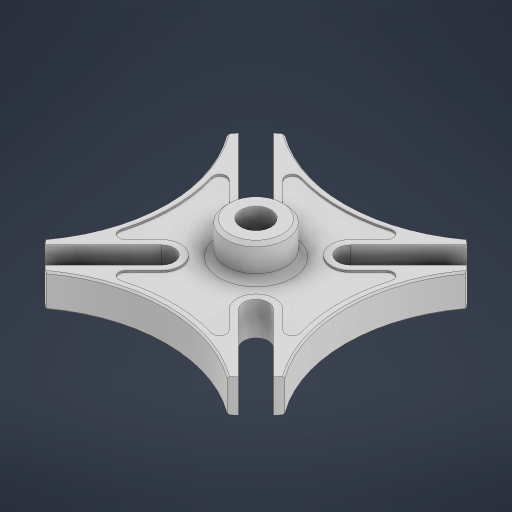
# Autodesk Inventor part: Malta cross
Saved by Autodesk Inventor 2023.2 (Build 272271000, 271)
## iProperties
Created: 2022-11-28
Part Number: Malta cross
Material: Generic
Document SubType Name: Modeling
Designer: iusti
Density: 1 g/cm^3
Appearance: Gunmetal - Antique Polished
Author: iusti
Autodesk Inventor part; units mm, degrees
ref_plane "YZ Plane" through (0, 0, 0) normal (1, 0, 0) x (0, 1, 0)
ref_plane "XZ Plane" through (0, 0, 0) normal (0, 1, 0) x (-1, 0, 0)
sketch "Sketch2" plane through (0, 0, 0) normal (0, 1, 0) x (-1, 0, 0)
  circle A0 centre (0, 0) radius 45 construction
  arc A1 (35.8767, 27.1636) -> (35.8767, -27.1636) centre (73, 0) ccw
  arc A2 (-27.1636, 35.8767) -> (27.1636, 35.8767) centre (0, 73) ccw
  arc A3 (-35.8767, -27.1636) -> (-35.8767, 27.1636) centre (-73, 0) ccw
  arc A4 (27.1636, -35.8767) -> (-27.1636, -35.8767) centre (0, -73) ccw
  circle A5 centre (0, 0) radius 20 construction
  line L0 (0, 0) -> (31.8198, -31.8198) construction
  line L1 (0, 0) -> (45, 0) construction
  arc A6 (16.7584, -11.5258) -> (11.5258, -16.7584) centre (14.1421, -14.1421) ccw
  line L2 (16.7584, -11.5258) -> (34.3284, -29.0958)
  line L3 (11.5258, -16.7584) -> (29.0958, -34.3284)
  arc A7 (34.3284, -29.0958) -> (35.8767, -27.1636) centre (0, 0) ccw
  arc A8 (27.1636, -35.8767) -> (29.0958, -34.3284) centre (0, 0) ccw
  arc A9 (11.5258, 16.7584) -> (16.7584, 11.5258) centre (14.1421, 14.1421) ccw
  line L4 (16.7584, 11.5258) -> (34.3284, 29.0958)
  line L5 (11.5258, 16.7584) -> (29.0958, 34.3284)
  arc A10 (29.0958, 34.3284) -> (27.1636, 35.8767) centre (0, 0) ccw
  arc A11 (35.8767, 27.1636) -> (34.3284, 29.0958) centre (0, 0) ccw
  arc A12 (-16.7584, 11.5258) -> (-11.5258, 16.7584) centre (-14.1421, 14.1421) ccw
  line L6 (-11.5258, 16.7584) -> (-29.0958, 34.3284)
  line L7 (-16.7584, 11.5258) -> (-34.3284, 29.0958)
  arc A13 (-34.3284, 29.0958) -> (-35.8767, 27.1636) centre (0, 0) ccw
  arc A14 (-27.1636, 35.8767) -> (-29.0958, 34.3284) centre (0, 0) ccw
  arc A15 (-11.5258, -16.7584) -> (-16.7584, -11.5258) centre (-14.1421, -14.1421) ccw
  line L8 (-16.7584, -11.5258) -> (-34.3284, -29.0958)
  line L9 (-11.5258, -16.7584) -> (-29.0958, -34.3284)
  arc A16 (-29.0958, -34.3284) -> (-27.1636, -35.8767) centre (0, 0) ccw
  arc A17 (-35.8767, -27.1636) -> (-34.3284, -29.0958) centre (0, 0) ccw
  point P0 (27.1636, 35.8767)
  point P1 (-27.1636, 35.8767)
  point P2 (-35.8767, 27.1636)
  point P3 (-27.1636, -35.8767)
  point P4 (35.8767, 27.1636)
  dimension "d14" = 40
  dimension "d7" = 90
  dimension "d8" = 46
  dimension "d9" = 73
  dimension "d12" = 360
  dimension "d15" = 45
  dimension "d16" = 7.4
  dimension "d19" = 360
  constraints: 36 point on circle, 20 end point, 17 centre point, 7 coincident, 2 symmetric about line, 1 equal length, 1 horizontal, 1 parallel, 1 point on line, 1 tangent, 1 vertical alignment, 77 other
  measures "d7" diameter of A0
  measures "d8" radius of A1
  measures "d9" distance of A1.centre point (0, 0)
  measures "d15" angle of L0 L1
  measures "d16" diameter of A6
extrude "Extrusion1" add sketch "Sketch2" along normal blind 10
sketch "Sketch3" plane through (0, 10, 0) normal (0, 1, 0) x (1, 0, 0)
  arc A0 (27.1636, -35.8767) -> (-27.1636, -35.8767) centre (0, -73) ccw projected
  line L0 (29.0958, -34.3284) -> (11.5258, -16.7584) projected
  arc A1 (16.7584, -11.5258) -> (11.5258, -16.7584) centre (14.1421, -14.1421) ccw projected
  line L1 (16.7584, -11.5258) -> (34.3284, -29.0958) projected
  arc A2 (35.8767, 27.1636) -> (35.8767, -27.1636) centre (73, 0) ccw projected
  line L2 (34.3284, 29.0958) -> (16.7584, 11.5258) projected
  arc A3 (11.5258, 16.7584) -> (16.7584, 11.5258) centre (14.1421, 14.1421) ccw projected
  line L3 (11.5258, 16.7584) -> (29.0958, 34.3284) projected
  arc A4 (-27.1636, 35.8767) -> (27.1636, 35.8767) centre (0, 73) ccw projected
  line L4 (-29.0958, 34.3284) -> (-11.5258, 16.7584) projected
  arc A5 (-16.7584, 11.5258) -> (-11.5258, 16.7584) centre (-14.1421, 14.1421) ccw projected
  line L5 (-16.7584, 11.5258) -> (-34.3284, 29.0958) projected
  arc A6 (-35.8767, -27.1636) -> (-35.8767, 27.1636) centre (-73, 0) ccw projected
  line L6 (-34.3284, -29.0958) -> (-16.7584, -11.5258) projected
  arc A7 (-11.5258, -16.7584) -> (-16.7584, -11.5258) centre (-14.1421, -14.1421) ccw projected
  line L7 (-11.5258, -16.7584) -> (-29.0958, -34.3284) projected
  line L8 (-15.5707, -23.6317) -> (-10.1116, -18.1726)
  arc A8 (-10.1116, -18.1726) -> (-18.1726, -10.1116) centre (-14.1421, -14.1421) ccw
  line L9 (-18.1726, -10.1116) -> (-23.6317, -15.5707)
  arc A9 (-26.9641, -13.5902) -> (-26.9641, 13.5902) centre (-73, 0) ccw
  line L10 (-23.6317, 15.5707) -> (-18.1726, 10.1116)
  arc A10 (-18.1726, 10.1116) -> (-10.1116, 18.1726) centre (-14.1421, 14.1421) ccw
  line L11 (-10.1116, 18.1726) -> (-15.5707, 23.6317)
  arc A11 (-13.5902, 26.9641) -> (13.5902, 26.9641) centre (0, 73) ccw
  line L12 (15.5707, 23.6317) -> (10.1116, 18.1726)
  arc A12 (10.1116, 18.1726) -> (18.1726, 10.1116) centre (14.1421, 14.1421) ccw
  line L13 (18.1726, 10.1116) -> (23.6317, 15.5707)
  arc A13 (26.9641, 13.5902) -> (26.9641, -13.5902) centre (73, 0) ccw
  line L14 (23.6317, -15.5707) -> (18.1726, -10.1116)
  arc A14 (18.1726, -10.1116) -> (10.1116, -18.1726) centre (14.1421, -14.1421) ccw
  line L15 (10.1116, -18.1726) -> (15.5707, -23.6317)
  arc A15 (13.5902, -26.9641) -> (-13.5902, -26.9641) centre (0, -73) ccw
  arc A16 (-15.5707, -23.6317) -> (-13.5902, -26.9641) centre (-14.1565, -25.0459) ccw
  arc A17 (-26.9641, -13.5902) -> (-23.6317, -15.5707) centre (-25.0459, -14.1565) ccw
  arc A18 (-23.6317, 15.5707) -> (-26.9641, 13.5902) centre (-25.0459, 14.1565) ccw
  arc A19 (-13.5902, 26.9641) -> (-15.5707, 23.6317) centre (-14.1565, 25.0459) ccw
  arc A20 (15.5707, 23.6317) -> (13.5902, 26.9641) centre (14.1565, 25.0459) ccw
  arc A21 (26.9641, 13.5902) -> (23.6317, 15.5707) centre (25.0459, 14.1565) ccw
  arc A22 (23.6317, -15.5707) -> (26.9641, -13.5902) centre (25.0459, -14.1565) ccw
  arc A23 (13.5902, -26.9641) -> (15.5707, -23.6317) centre (14.1565, -25.0459) ccw
  point P0 (-22.5835, -30.6446)
  point P1 (-30.6446, -22.5835)
  point P2 (-30.6446, 22.5835)
  point P3 (-22.5835, 30.6446)
  point P4 (22.5835, 30.6446)
  point P5 (30.6446, 22.5835)
  point P6 (30.6446, -22.5835)
  point P7 (22.5835, -30.6446)
  dimension "d23" = 2
  dimension "d24" = 2
  constraints: 40 point on circle, 16 centre point, 16 end point, 16 tangent, 8 point on line, 7 equal radius, 15 other
  measures "d23" radial gap between concentric circles of A0 A15
  measures "d24" radius of A16
extrude "Extrusion2" cut sketch "Sketch3" against normal blind 0.5
ref_plane "Work Plane1" through (0, 5, 0) normal (0, 1, 0) x (1, 0, 0)
mirror "Mirror1" about plane through (0, 5, 0) normal (0, 1, 0) of "Extrusion2"
sketch "Sketch4" plane through (0, 9.5, 0) normal (0, 1, 0) x (1, 0, 0)
  circle A0 centre (0, 0) radius 9
  dimension "d27" = 18
  constraints: 1 centre point, 1 coincident
  measures "d27" diameter of A0
extrude "Extrusion3" add sketch "Sketch4" along normal blind 10
sketch "Sketch5" plane through (0, 19.5, 0) normal (0, 1, 0) x (1, 0, 0)
  circle A0 centre (0, 0) radius 9 projected
  constraints: 1 coincident
hole "Hole1" at (0, 19.5, 0) direction (0, -1, 0) diameter 9 end through all
chamfer "Chamfer1" distance 1 angle 45 1 edges at (-9, 19.5, 0)
fillet "Fillet1" radius 2 1 edges at (-9, 9.5, 0)
chamfer "Chamfer3" distance 0.5 angle 45 8 edges at (-27, 10, 0) (0, 10, -27) (27, 10, 0) (0, 10, 27) (0, 0, 27) (-27, 0, 0) (0, 0, -27) (27, 0, 0)
body "Solid1"
